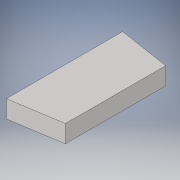
# Autodesk Inventor part: InsertTest1
Saved by Autodesk Inventor 2018 (Build 220112000, 112)
## iProperties
Created: 2019-03-20
Part Number: InsertTest1
Material: Generic
Document SubType Name: Modeling
Designer: 871357
Density: 1 g/cm^3
Appearance: Default
Author: 871357
Autodesk Inventor part; units mm, degrees
ref_plane "YZ Plane" through (0, 0, 0) normal (1, 0, 0) x (0, 1, 0)
ref_plane "XZ Plane" through (0, 0, 0) normal (0, 1, 0) x (-1, 0, 0)
ref_plane "XY Plane" through (0, 0, 0) normal (0, 0, 1) x (1, 0, 0)
sketch "Sketch1" plane through (0, 0, 0) normal (0, 1, 0) x (-1, 0, 0)
  line L0 (-3.587, 3.9917) -> (-3.587, -10.4863)
  line L1 (-3.587, -10.4863) -> (3.779, -11.6293)
  line L2 (3.779, -11.6293) -> (3.779, 5.1347)
  line L3 (3.779, 5.1347) -> (-3.587, 3.9917)
  point P0 (0, 0)
  dimension "d0" = 16.764
  dimension "d1" = 14.478
  dimension "d2" = 7.366
  constraints: 8 end point, 1 equal length, 1 parallel, 1 vertical
  measures "d0" distance of L1.end L2.end
  measures "d1" distance of L0.start L0.end
  measures "d2" distance between parallel lines of L0 L2
extrude "Extrusion1" add sketch "Sketch1" along normal blind 2.54
body "Solid1"
